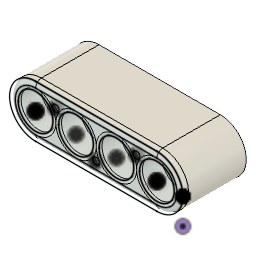
Nixie Clock for 3D Print v1.1 (Autodesk Fusion 360 design; units mm, degrees)
Autodesk Fusion 360 part; units mm, degrees
sketch "Geometry" plane through (0, 0, 0) normal (0, 0, 1) x (1, 0, 0)
  arc A0 (22.5, 45) -> (22.5, 0) centre (22.5, 22.5) ccw
  arc A1 (127.5, 0) -> (127.5, 45) centre (127.5, 22.5) ccw
  line L0 (22.5, 45) -> (127.5, 45)
  line L1 (22.5, 0) -> (127.5, 0)
  arc A2 (127.5, 5) -> (127.5, 40) centre (127.5, 22.5) ccw
  line L2 (22.5, 40) -> (127.5, 40)
  arc A3 (22.5, 40) -> (22.5, 5) centre (22.5, 22.5) ccw
  line L3 (22.5, 5) -> (127.5, 5)
  circle A4 centre (22.5, 22.5) radius 15
  circle A5 centre (127.5, 22.5) radius 15
  circle A6 centre (57.5, 22.5) radius 15
  circle A7 centre (92.5, 22.5) radius 15
  circle A8 centre (75, 11.5) radius 2.85
  circle A9 centre (40, 33.5) radius 2.85
  circle A10 centre (110, 33.5) radius 2.85
  point P0 (0, 22.5)
  dimension "d19" = 105
  dimension "d21" = 30
  dimension "d22" = 30
  dimension "d23" = 30
  dimension "d24" = 35
  dimension "d25" = 30
  dimension "d26" = 35
  dimension "d27" = 11
  dimension "d28" = 11
  dimension "d29" = 5.7
  dimension "d30" = 5.7
  dimension "d31" = 5.7
  dimension "d32" = 11
  dimension "d33" = 17.5
  dimension "d34" = 17.5
  dimension "d35" = 17.5
  dimension "d44" = 35
  dimension "d45" = 5
  constraint tangent A1 L0
  constraint tangent A1 L1
  constraint tangent A0 L1
  constraint horizontal L0
  constraint tangent A0 L0
  constraint coincident origin L1
  constraint midpoint A0 P0
  constraint vertical origin P0
  constraint concentric A0 A4
  constraint concentric A1 A5
  constraint horizontal A0.centre A6.centre
  constraint horizontal A6.centre A7.centre
  measures "d19" distance of A0.centre A1.centre
  measures "d21" diameter of A4
  measures "d22" diameter of A5
  measures "d23" diameter of A6
  measures "d24" distance of A0.centre A6.centre
  measures "d25" diameter of A7
  measures "d26" distance of A6.centre A7.centre
  measures "d27" vertical distance of A6.centre A8.centre
  measures "d28" vertical distance of A0.centre A9.centre
  measures "d29" diameter of A10
  measures "d30" diameter of A8
  measures "d31" diameter of A9
  measures "d32" vertical distance of A7.centre A10.centre
  measures "d33" horizontal distance of A0.centre A9.centre
  measures "d34" horizontal distance of A1.centre A10.centre
  measures "d35" horizontal distance of A6.centre A8.centre
  measures "d44" distance of L2 L3
extrude "Paroi Boite" add sketch "Geometry" along normal blind 55 contours A0 A1 L0 L1
extrude "Percage Nixies" add sketch "Geometry" along normal blind 20 contours A2 L2 A3 L3 | A4 | A5 | A6 | A7 | A8 | A9 | A10
extrude "Inserts" cut sketch "Geometry" against normal blind 9 from surface at 20 contours A8 | A9 | A10
extrude "Extrude7" cut sketch "Geometry" along normal up to surface (20 mm away) draft 1.5 contours A4 | A5 | A6 | A7
ref_plane "WorkPlane1" through (0, 22.5, 0) normal (0, 1, 0) x (0, 0, 1)
ref_plane "WorkPlane2" through (40, 0, 0) normal (1, 0, 0) x (0, 1, 0)
fillet "Fillet1" radius 5 4 edges at (150, 22.5, 0) (75, 45, 0) (0, 22.5, 0) (75, 0, 0)
fillet "Fillet1" radius 2.43 4 edges at (8.5151, 17.0758, 0) (43.5151, 17.0758, 0) (78.5151, 17.0758, 0) (113.5151, 17.0758, 0)
sketch "Bottom" plane through (0, 0, 0) normal (0, -1, 0) x (1, 0, 0)
  line L0 (127.5, 5) -> (127.5, 55)
  line L1 (127.5, 55) -> (22.5, 55)
  line L2 (22.5, 55) -> (22.5, 5)
  circle A0 centre (119.5, 13) radius 6.5
  circle A1 centre (30.5, 13) radius 6.5
  line L3 (75, 5) -> (100, 30)
  line L4 (100, 30) -> (75, 55)
  line L5 (75, 5) -> (50, 30)
  line L6 (50, 30) -> (75, 55)
  line L7 (92.6777, 30) -> (75, 47.6777)
  line L8 (75, 47.6777) -> (69.461, 42.1387)
  line L9 (69.461, 42.1387) -> (75.7071, 35.8926)
  line L10 (75.7071, 35.8926) -> (70.1681, 30.3536)
  line L11 (70.1681, 30.3536) -> (75.3536, 25.1681)
  line L12 (75.3536, 25.1681) -> (80.8926, 30.7071)
  line L13 (80.8926, 30.7071) -> (81.9532, 29.6464)
  line L14 (81.9532, 29.6464) -> (76.4142, 24.1074)
  line L15 (76.4142, 24.1074) -> (81.5997, 18.922)
  line L16 (81.5997, 18.922) -> (92.6777, 30)
  line L17 (80.539, 17.8613) -> (68.0468, 30.3536)
  line L18 (68.0468, 30.3536) -> (73.5858, 35.8926)
  line L19 (73.5858, 35.8926) -> (68.4003, 41.078)
  line L20 (68.4003, 41.078) -> (57.3223, 30)
  line L21 (57.3223, 30) -> (75, 12.3223)
  line L22 (75, 12.3223) -> (80.539, 17.8613)
  line L23 (55.201, 30) -> (75, 49.799)
  line L24 (75, 49.799) -> (94.799, 30)
  line L25 (94.799, 30) -> (75, 10.201)
  line L26 (75, 10.201) -> (55.201, 30)
  line L27 (22.5, 5) -> (127.5, 5)
  dimension "d51" = 13
  dimension "d52" = 8
  dimension "d61" = 8
  dimension "d78" = 1.5
  dimension "d79" = 1.5
  dimension "d80" = 1.5
  dimension "d81" = 1.5
  dimension "d82" = 25
  dimension "d84" = 7.8333
  dimension "d85" = 7.3333
  dimension "d86" = 7.3333
  dimension "d87" = 7.8333
  dimension "d88" = 25
  dimension "d89" = 1.5
  dimension "d90" = 1.5
  dimension "d91" = 1.5
  dimension "d92" = 1.5
  dimension "d93" = 13
  constraint midpoint L1 L4.end
  constraint perpendicular L5 L6
  constraint perpendicular L3 L4
  constraint perpendicular L3 L5
  constraint coincident L3.start L5.start
  constraint horizontal L3.end L5.end
  constraint perpendicular L7 L8
  constraint perpendicular L7 L10
  constraint perpendicular L10 L11
  constraint perpendicular L11 L12
  constraint perpendicular L11 L14
  constraint perpendicular L16 L17
  constraint perpendicular L17 L18
  constraint parallel L15 L19
  constraint perpendicular L19 L20
  constraint parallel L3 L22
  constraint parallel L3 L16
  constraint parallel L4 L7
  constraint parallel L6 L20
  constraint parallel L5 L21
  constraint parallel L4 L13
  constraint collinear L8 L20
  constraint collinear L11 L15
  constraint parallel L4 L9
  constraint collinear L16 L22
  constraint horizontal L3.end L7.start
  constraint vertical L3.start L21.end
  constraint collinear L9 L13
  constraint perpendicular L21 L23
  constraint perpendicular L6 L24
  constraint perpendicular L21 L25
  constraint parallel L5 L26
  measures "d51" diameter of A0
  measures "d52" distance of L0 A0.centre
  measures "d61" distance of L2 A1.centre
  measures "d78" distance of L9 L19
  measures "d79" distance of L10 L18
  measures "d80" distance of L12 L14
  measures "d81" distance of L15 L17
  measures "d82" distance of L7 L21
  measures "d84" distance of L17.start L21.end
  measures "d85" distance of L14.end L15.end
  measures "d86" distance of L10.end L11.end
  measures "d87" distance of L7.end L8.end
  measures "d88" distance of L20 L22
  measures "d89" distance of L20 L23
  measures "d90" distance of L21 L26
  measures "d91" distance of L22 L25
  measures "d92" distance of L7 L24
  measures "d93" diameter of A1
extrude "Extrude5" cut sketch "Bottom" against normal blind 1 contours L23 L24 L25 L26
ref_plane "WorkPlane3" through (101.25, -2.5, 30) normal (0, -1, 0) x (1, 0, 0)
sketch "Sketch5" plane through (0, -2.5, 0) normal (0, -1, 0) x (-1, 0, 0)
  circle A0 centre (-30.5, -13) radius 6.5
  circle A1 centre (-119.5, -13) radius 6.5
  line L0 (-30.5, -19.5) -> (-119.5, -19.5)
  constraint coincident A0 L0.start
  constraint coincident A1 L0.end
  constraint tangent A1 L0
  constraint tangent A0 L0
ref_plane "WorkPlane4" through (30.5, -2.5, 19.5) normal (0, -0.99753, 0.070249) x (1, 0, 0)
sketch "Sketch6" plane through (0, -3.8541, 0.2714) normal (0, -0.99753, 0.070249) x (1, 0, 0)
  circle A0 centre (30.5, 12.9679) radius 6.5
  circle A1 centre (119.5, 12.9679) radius 6.5
  point P0 (30.5, 12.9679)
  point P1 (119.5, 12.9679)
  dimension "d95" = 13
  dimension "d96" = 13
  constraint coincident P0 A0.centre
  constraint coincident P1 A1.centre
  measures "d95" diameter of A0
  measures "d96" diameter of A1
extrude "Extrude6" cut sketch "Sketch6" against normal blind 3.5
equation "d79 = d78"
equation "d80 = d78"
equation "d81 = d78"
equation "d84 = ( d82 - d81 ) / 3"
equation "d85 = d84 - d78 / 3"
equation "d86 = d84 - d78 / 3"
equation "d87 = d84"
equation "d88 = d82"
equation "d89 = d78"
equation "d90 = d78"
equation "d91 = d78"
equation "d92 = d78"
named bodies: "Nixie Clock Case"
